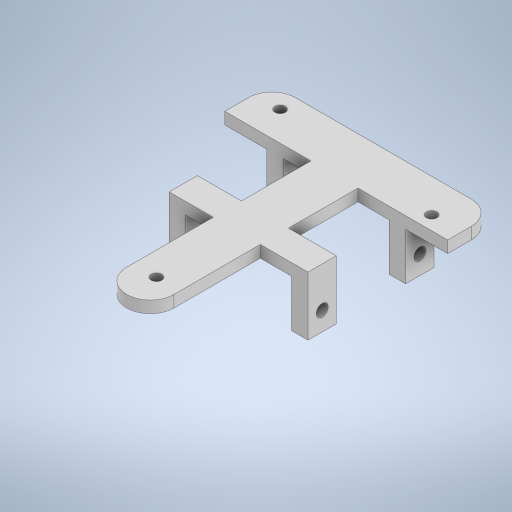
# Autodesk Inventor part: TALLER_SkyhopperMount
Saved by Autodesk Inventor 2023 (Build 270158000, 158)
## iProperties
Created: 2022-06-29
Part Number: TALLER_SkyhopperMount
Material: Generic
Document SubType Name: Modeling
Designer: jaspe
Density: 1 g/cm^3
Appearance: Default
Author: jaspe
Autodesk Inventor part; units mm, degrees
ref_plane "YZ Plane" through (0, 0, 0) normal (1, 0, 0) x (0, 1, 0)
ref_plane "XZ Plane" through (0, 0, 0) normal (0, 1, 0) x (-1, 0, 0)
ref_plane "XY Plane" through (0, 0, 0) normal (0, 0, 1) x (1, 0, 0)
sketch "Sketch1" plane through (0, 0, 0) normal (0, 1, 0) x (-1, 0, 0)
  line L0 (20.0829, 44.2754) -> (-39.9171, 44.2754)
  line L1 (-39.9171, 44.2754) -> (-39.9171, -37.0246)
  line L2 (-39.9171, -37.0246) -> (20.0829, -37.0246)
  line L3 (20.0829, -37.0246) -> (20.0829, 44.2754)
  point P0 (0, 0)
  dimension "d0" = 60
  dimension "d1" = 81.3
  constraints: 8 end point, 2 parallel, 1 horizontal, 1 perpendicular
  measures "d0" distance of L0.start L0.end
  measures "d1" distance of L2.end L0.start
extrude "Extrusion1" add sketch "Sketch1" along normal blind 3.175
sketch "Sketch8" plane through (0, 0, 0) normal (0, -1, 0) x (1, 0, 0)
  circle A0 centre (9.4171, 36.2754) radius 1.397
  circle A1 centre (-13.0829, -19.5246) radius 1.397
  circle A2 centre (31.9171, -15.3246) radius 1.397
  line L0 (39.9171, 44.2754) -> (39.9171, -37.0246) projected
  line L1 (39.9171, -37.0246) -> (-20.0829, -37.0246) projected
  point P0 (0, 0)
  point P1 (39.9171, 42.2754)
  point P2 (39.9171, -35.0246)
  point P3 (37.9171, -37.0246)
  point P4 (-18.0829, -37.0246)
  dimension "d76" = 8
  dimension "d77" = 21.7
  dimension "d78" = 4.2
  dimension "d79" = 45
  dimension "d80" = 22.5
  dimension "d81" = 51.6
  dimension "d97" = 2.794
  constraints: 3 centre point, 2 equal radius
  measures "d76" distance from line of L0 A2.centre
  measures "d77" distance from line of L1 A2.centre
  measures "d78" vertical distance of A1.centre A2.centre
  measures "d79" horizontal distance of A2.centre A1.centre
  measures "d80" horizontal distance of A0.centre A2.centre
  measures "d81" vertical distance of A0.centre A2.centre
  measures "d97" diameter of A2
extrude "Extrusion6" cut sketch "Sketch8" against normal blind 4
sketch "Sketch9" plane through (0, 0, 0) normal (0, -1, 0) x (1, 0, 0)
  line L0 (39.9171, -37.0246) -> (-20.0829, -37.0246) projected
  line L1 (-20.0829, -24.3246) -> (39.9171, -24.3246)
  line L2 (39.9171, -24.3246) -> (39.9171, -37.0246)
  line L3 (39.9171, -37.0246) -> (-20.0829, -37.0246)
  line L4 (-20.0829, -37.0246) -> (-20.0829, -24.3246)
  line L5 (39.9171, 44.2754) -> (39.9171, -37.0246) projected
  line L6 (39.9171, -11.6246) -> (15.7671, -11.6246)
  line L7 (15.7671, -11.6246) -> (15.7671, 7.0444)
  line L8 (15.7671, 7.0444) -> (39.9171, 7.0444)
  line L9 (39.9171, 7.0444) -> (39.9171, -11.6246)
  line L10 (-20.0829, -11.6246) -> (3.0671, -11.6246)
  line L11 (3.0671, -11.6246) -> (3.0671, 7.0444)
  line L12 (3.0671, 7.0444) -> (-20.0829, 7.0444)
  line L13 (-20.0829, 7.0444) -> (-20.0829, -11.6246)
  circle A0 centre (9.4171, 36.2754) radius 1.397 construction
  line L14 (9.4171, 36.2754) -> (9.4171, 34.8784) construction
  line L15 (-20.0829, 44.2754) -> (39.9171, 44.2754) construction
  line L16 (-20.0829, -37.0246) -> (-20.0829, 44.2754) projected
  line L17 (-20.0829, -37.0246) -> (-20.0829, 44.2754) projected
  line L18 (-20.0829, 44.2754) -> (3.0671, 44.2754)
  line L19 (3.0671, 44.2754) -> (3.0671, 14.6644)
  line L20 (3.0671, 14.6644) -> (-20.0829, 14.6644)
  line L21 (-20.0829, 14.6644) -> (-20.0829, 44.2754)
  line L22 (-20.0829, 44.2754) -> (39.9171, 44.2754) projected
  line L23 (15.7671, 14.6644) -> (39.9171, 14.6644)
  line L24 (39.9171, 14.6644) -> (39.9171, 44.2754)
  line L25 (39.9171, 44.2754) -> (15.7671, 44.2754)
  line L26 (15.7671, 44.2754) -> (15.7671, 14.6644)
  line L27 (-20.0829, 14.6644) -> (-8.7773, 14.6644)
  line L28 (-8.7773, 14.6644) -> (-8.7773, 7.0444)
  line L29 (-8.7773, 7.0444) -> (-20.0829, 7.0444)
  line L30 (-20.0829, 7.0444) -> (-20.0829, 14.6644)
  line L31 (39.9171, 14.6644) -> (28.6115, 14.6644)
  line L32 (28.6115, 14.6644) -> (28.6115, 7.0444)
  line L33 (28.6115, 7.0444) -> (39.9171, 7.0444)
  line L34 (39.9171, 7.0444) -> (39.9171, 14.6644)
  line L35 (9.9171, 44.2754) -> (9.9171, -37.0246) construction
  point P0 (0, 0)
  point P1 (3.0671, -2.2901)
  point P2 (39.9171, 7.0444)
  point P3 (-8.7773, 14.6644)
  point P4 (28.6115, 14.6644)
  dimension "d98" = 12.7
  dimension "d99" = 12.7
  dimension "d100" = 12.7
  dimension "d142" = 18.669
  dimension "d143" = 7.62
  dimension "d144" = 37.3888
  constraints: 60 end point, 14 parallel, 7 collinear, 7 horizontal, 7 perpendicular, 3 midpoint, 3 point on line, 1 vertical, 1 vertical alignment, 3 other
  measures "d98" distance between parallel lines of L1 L10
  measures "d99" distance from line of point (3.067, -2.29) L7
  measures "d100" distance between parallel lines of L0 L1
  measures "d142" distance between parallel lines of L12 L10
  measures "d143" distance between parallel lines of L20 L12
  measures "d144" distance between parallel lines of L32 L28
sketch "Sketch11" plane through (0, 3.175, 0) normal (0, 1, 0) x (1, 0, 0)
  line L0 (3.0671, 11.6246) -> (-20.0829, 11.6246) projected
  line L1 (-8.7773, 19.2446) -> (-4.3323, 19.2446)
  line L2 (-4.3323, 19.2446) -> (-4.3323, 11.6246)
  line L3 (-4.3323, 11.6246) -> (-8.7773, 11.6246)
  line L4 (-8.7773, 11.6246) -> (-8.7773, 19.2446)
  line L5 (39.9171, 11.6246) -> (15.7671, 11.6246) projected
  line L6 (24.1665, 19.2446) -> (28.6115, 19.2446)
  line L7 (28.6115, 19.2446) -> (28.6115, 11.6246)
  line L8 (28.6115, 11.6246) -> (24.1665, 11.6246)
  line L9 (24.1665, 11.6246) -> (24.1665, 19.2446)
  line L10 (39.9171, 24.3246) -> (-20.0829, 24.3246) construction
  line L11 (9.9171, 24.3246) -> (9.9171, -44.2754) construction
  line L12 (-20.0829, -44.2754) -> (39.9171, -44.2754) construction
  point P0 (0, 0)
  dimension "d115" = 28.4988
  dimension "d116" = 7.62
  dimension "d117" = 4.445
  constraints: 18 end point, 4 parallel, 3 point on line, 2 horizontal, 2 midpoint, 2 perpendicular, 1 collinear, 1 other
  measures "d115" distance between parallel lines of L9 L2
  measures "d116" distance of L3.end L1.start
  measures "d117" distance of L1.start L1.end
extrude "Extrusion9" add sketch "Sketch11" against normal blind 15.875
sketch "Sketch12" plane through (28.6115, 3.175, -11.6246) normal (1, 0, 0) x (0, 0, 1)
  line L0 (-7.62, 15.875) -> (0, 15.875) projected
  line L1 (-7.62, 3.175) -> (-7.62, 15.875) projected
  point P0 (11.6246, 3.175)
  point P1 (-3.81, 10.795)
  point P2 (7.62, 0)
  dimension "d130" = 5.08
  dimension "d148" = 3.81
  constraints: 1 other
  measures "d130" distance from line of L0 point (-3.81, 10.795)
hole "Hole1" at (28.6115, -7.62, -15.4346) direction (-1, 0, 0) diameter 3.175 depth 37.3888
pattern_linear "Rectangular Pattern1" count 2 spacing 26.289 along (0, 0, 1) of "Extrusion9", "Hole1"
extrude "Extrusion10" cut sketch "Sketch9" against normal blind 25.4 contours L0 L4 L1 L2 | L6 L7 L8 L5 | L13 L12 L11 L10 | L8 L32 L23 L5 | L16 L20 L28 L12 | L23 L26 L22 L5 | L16 L18 L19 L20
fillet "Fillet2" radius 6.35 4 edges at (3.0671, 1.5875, 44.2754) (15.7671, 1.5875, 44.2754) (-20.0829, 1.5875, -24.3246) (39.9171, 1.5875, -24.3246)
body "Solid1"
